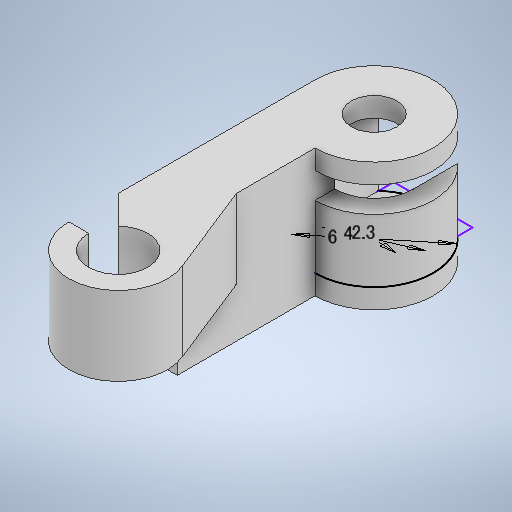
# Autodesk Inventor part: srod1.1
Saved by Autodesk Inventor 2025 (Build 290162000, 162)
## iProperties
Created: 2024-07-27
Part Number: srod1.1
Material: 一般
Document SubType Name: Modeling
Designer: Saigusa
Density: 1 g/cm^3
Appearance: 既定
Author: Saigusa
Autodesk Inventor part; units mm, degrees
ref_plane "YZ Plane" through (0, 0, 0) normal (1, 0, 0) x (0, 1, 0)
ref_plane "XZ Plane" through (0, 0, 0) normal (0, 1, 0) x (-1, 0, 0)
ref_plane "XY Plane" through (0, 0, 0) normal (0, 0, 1) x (1, 0, 0)
sketch "スケッチ1" plane through (0, 0, 0) normal (0, 1, 0) x (-1, 0, 0)
  circle A0 centre (0, 0) radius 1.15
  circle A1 centre (0, 0) radius 2
  circle A2 centre (0, 0) radius 3
  line L0 (0, 0) -> (0, 3)
  line L1 (-2, 0) -> (2, 0)
  line L2 (2, 0) -> (2, -3)
  line L3 (2, -3) -> (-2, -3)
  line L4 (-2, -3) -> (-2, 0)
  line L5 (0, 0) -> (3, 0)
  line L6 (3, 0) -> (3, 3)
  line L7 (3, 3) -> (0, 3)
  line L8 (0, 3) -> (0, 0)
  point P0 (-2, -2.2361)
  point P1 (0, 2)
  point P2 (2, -2.2361)
  dimension "d1" = 4
  dimension "d2" = 6
  dimension "d0" = 2.3
  constraints: 18 end point, 4 parallel, 3 coincident, 2 horizontal, 2 perpendicular, 1 centre point, 1 vertical, 6 other
  measures "d0" diameter of A0
extrude "押し出し1" add sketch "スケッチ1" along normal blind 3.2 contours A1 L4 A2 L0
extrude "押し出し2" add sketch "スケッチ1" along normal blind 4.5 contours L5 A2 L2 | A1 L0 A2 L5 | A2 L7 L6
extrude "押し出し3" add sketch "スケッチ1" against normal blind 1 contours L1 A1 A0 | A0 L0 A1 L1 | A0 L1 A1 L0 | L2 A2 L4 A1 | L5 A2 L2 | A1 L0 A2 L5 | A1 L4 A2 L0 | A2 L7 L6
sketch "スケッチ2" plane through (0, 4.5, 0) normal (0, 1, 0) x (1, 0, 0)
  circle A0 centre (0, 0) radius 1.15
  circle A1 centre (0, 0) radius 2
  circle A2 centre (0, 0) radius 3
  line L0 (0, 0) -> (-3, 0)
  line L1 (-3, 0) -> (-3, -3)
  line L2 (-3, -3) -> (0, -3)
  line L3 (0, -3) -> (0, 0)
  dimension "d9" = 2.3
  dimension "d10" = 4
  dimension "d11" = 6
  constraints: 8 end point, 3 centre point, 3 coincident, 2 parallel, 1 horizontal, 1 perpendicular
  measures "d9" diameter of A0
  measures "d10" diameter of A1
  measures "d11" diameter of A2
extrude "押し出し4" add sketch "スケッチ2" along normal blind 1 contours A0 L0 A1 L3 | A0 L3 A1 L0 | L0 A2 L3 A1 | A1 L3 A2 L0 | A2 L2 L1
sketch "スケッチ3" plane through (-3, -1, 3) normal (0, 0, 1) x (1, 0, 0)
  line L0 (0, 6.5) -> (0, 0) projected
  line L1 (3, 5.5) -> (3, 6.5) projected
  line L2 (0, 0) -> (3, 0)
  line L3 (3, 0) -> (3, 6.5)
  line L4 (3, 6.5) -> (0, 6.5)
  line L5 (0, 6.5) -> (0, 0)
  point P0 (3, 1)
  constraints: 8 end point, 2 parallel, 1 horizontal, 1 perpendicular
extrude "押し出し5" add sketch "スケッチ3" along normal blind 7
sketch "スケッチ4" plane through (-3, -1, 10) normal (0, 0, 1) x (1, 0, 0)
  line L0 (4.15, 0) -> (1.85, 0) projected
  line L1 (3, 0) -> (1.5, 0)
  line L2 (1.5, 0) -> (1.5, 1.5)
  line L3 (1.5, 1.5) -> (3, 1.5)
  line L4 (3, 1.5) -> (3, 0)
  point P0 (3, 1)
  dimension "d16" = 1.5
  dimension "d17" = 1.5
  constraints: 8 end point, 2 parallel, 1 horizontal, 1 midpoint, 1 perpendicular
  measures "d16" distance of L2.end L3.end
  measures "d17" distance of L1.end L2.end
hole "穴1" at (-1.5, 0.5, 10) direction (0, 0, -1) diameter 1 end through all
sketch "スケッチ5" plane through (0, 3.2, 3) normal (1, 0, 0) x (0, 0, -1)
  point P0 (3, -3.2)
sketch "スケッチ6" plane through (0, 5.5, 0) normal (0, 1, 0) x (1, 0, 0)
  line L0 (-3, -10) -> (0, -10) projected
  line L1 (-3, -10) -> (2, -10)
  line L2 (2, -10) -> (2, -15)
  line L3 (2, -15) -> (-3, -15)
  line L4 (-3, -15) -> (-3, -10)
  line L5 (2, -10) -> (-0.5, -10)
  line L6 (-0.5, -10) -> (-0.5, -12.5)
  line L7 (-0.5, -12.5) -> (2, -12.5)
  line L8 (2, -12.5) -> (2, -10)
  circle A0 centre (-0.5, -12.5) radius 2.5
  circle A1 centre (-0.5, -12.5) radius 1.5
  line L9 (-0.5, -12.5) -> (-3, -10)
  line L10 (-0.5, -12.5) -> (-3, -12.5)
  line L11 (0, -3) -> (0, -10) projected
  line L12 (-3, -10) -> (0, -10)
  line L13 (0, -10) -> (0, -7)
  line L14 (0, -7) -> (-3, -7)
  line L15 (-3, -7) -> (-3, -10)
  line L16 (0, -7) -> (1.8225, -11.5748)
  point P0 (0, 0)
  point P1 (-2, -12.5)
  point P2 (-1.5607, -11.4393)
  dimension "d25" = 5
  dimension "d26" = 5
  dimension "d27" = 2.5
  dimension "d28" = 2.5
  dimension "d29" = 3
  dimension "d30" = 3
  constraints: 30 end point, 6 parallel, 3 horizontal, 3 perpendicular, 2 centre point, 2 coincident, 2 point on circle, 1 midpoint, 1 point on line, 1 tangent
  measures "d25" distance of L2.end L3.end
  measures "d26" distance of L1.end L2.end
  measures "d27" distance of L7.end L6.end
  measures "d28" distance of L6.end L5.end
  measures "d29" diameter of A1
  measures "d30" distance of L13.end L12.end
extrude "押し出し6" add sketch "スケッチ6" against normal blind 4 contours L0 A0 L9 | A0 L7 A1 L6 | L0 L1 L16 A0 | L6 A1 L9 A0 | L10 A1 L7 A0 | L11 L16 L1
